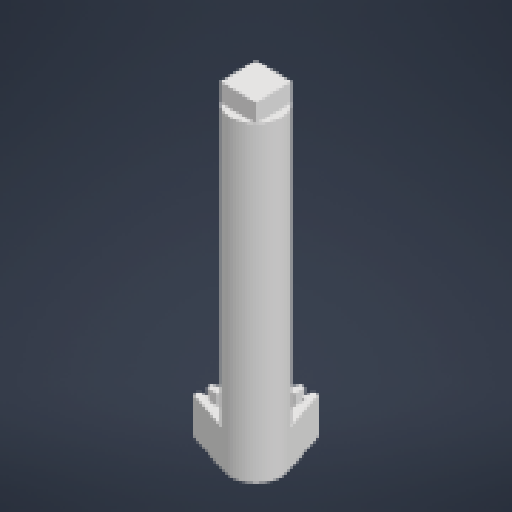
# Autodesk Inventor part: LegV2
Saved by Autodesk Inventor 2026 (Build 300175050, 175E)
## iProperties
Created: 2026-05-02
Part Number: LegV2
Material: Generic
Document SubType Name: Modeling
Designer: sniel
Density: 1 g/cm^3
Appearance: Default
Author: sniel
Autodesk Inventor part; units mm, degrees
ref_plane "YZ Plane" through (0, 0, 0) normal (1, 0, 0) x (0, 1, 0)
ref_plane "XZ Plane" through (0, 0, 0) normal (0, 1, 0) x (-1, 0, 0)
ref_plane "XY Plane" through (0, 0, 0) normal (0, 0, 1) x (1, 0, 0)
sketch "Sketch1" plane through (0, 0, 0) normal (0, 1, 0) x (-1, 0, 0)
  line L0 (0, 0) -> (10, 0)
  line L1 (0, 10) -> (0, 0)
  line L2 (10, 10) -> (0, 10)
  line L3 (10, 0) -> (10, 10)
  line L4 (0, 10) -> (0.05, 10)
  line L5 (0.05, 10) -> (0.05, 9.95)
  line L6 (0.05, 9.95) -> (0, 9.95)
  line L7 (0, 9.95) -> (0, 10)
  line L8 (10, 0) -> (9.95, 0)
  line L9 (9.95, 0) -> (9.95, 0.05)
  line L10 (9.95, 0.05) -> (10, 0.05)
  line L11 (10, 0.05) -> (10, 0)
  line L12 (0.05, 9.95) -> (9.95, 9.95)
  line L13 (9.95, 9.95) -> (9.95, 0.05)
  line L14 (9.95, 0.05) -> (0.05, 0.05)
  line L15 (0.05, 0.05) -> (0.05, 9.95)
  point P0 (0, 0)
  dimension "d0" = 0.05
  dimension "d1" = 0.05
  dimension "d2" = 0.05
  dimension "d3" = 0.05
  constraints: 32 end point, 6 parallel, 3 horizontal, 3 perpendicular
  measures "d0" distance of L5.end L6.end
  measures "d1" distance of L4.end L5.end
  measures "d2" distance of L9.end L10.end
  measures "d3" distance of L8.end L9.end
extrude "Extrusion1" add sketch "Sketch1" along normal blind 5 contours L14 L15 L12 L13
sketch "Sketch2" plane through (0, 0, 0) normal (0, -1, 0) x (1, 0, 0)
  line L0 (-0.05, 0.05) -> (-9.95, 0.05)
  line L1 (-0.05, 9.95) -> (-0.05, 0.05)
  line L2 (-9.95, 9.95) -> (-0.05, 9.95)
  line L3 (-9.95, 0.05) -> (-9.95, 9.95)
  line L4 (-0.05, 5) -> (-9.95, 5)
  circle A0 centre (-5, 5) radius 7.0004
  point P0 (0, 0)
  constraints: 10 end point, 3 midpoint, 3 other
extrude "Extrusion2" add sketch "Sketch2" along normal blind 85
sketch "Sketch4" plane through (-5, -85, 5) normal (0, -1, 0) x (1, 0, 0)
  circle A0 centre (0, 0) radius 7.0004
  circle A1 centre (0, 0) radius 7.0004 projected
  line L0 (0, -7.0004) -> (0, -12)
  line L1 (-2.5, -9.5) -> (2.5, -9.5)
  line L2 (2.5, -9.5) -> (2.5, -14.5)
  line L3 (2.5, -14.5) -> (-2.5, -14.5)
  line L4 (-2.5, -14.5) -> (-2.5, -9.5)
  line L5 (-2.5, -9.5) -> (2.5, -14.5) construction
  line L6 (2.5, -9.5) -> (-2.5, -14.5) construction
  line L7 (-7.0004, 0.0004) -> (-12.0004, 0.0004)
  line L8 (-9.5004, 2.5004) -> (-14.5004, 2.5004)
  line L9 (-14.5004, 2.5004) -> (-14.5004, -2.4996)
  line L10 (-14.5004, -2.4996) -> (-9.5004, -2.4996)
  line L11 (-9.5004, -2.4996) -> (-9.5004, 2.5004)
  line L12 (-9.5004, 2.5004) -> (-14.5004, -2.4996) construction
  line L13 (-14.5004, 2.5004) -> (-9.5004, -2.4996) construction
  line L14 (-9.5004, -2.4996) -> (-9.5004, -4.9996)
  line L15 (-14.5004, 2.5004) -> (-2.2357, 6.6338)
  line L16 (-14.5004, -2.4996) -> (-2.236, -6.6336)
  line L17 (-2.5, -14.5) -> (-6.6337, -2.2359)
  line L18 (2.5, -14.5) -> (6.6337, -2.2359)
  point P0 (5, -5)
  point P1 (-12.0004, 0.0004)
  point P2 (6.6337, -2.2359)
  point P3 (-2.2357, 6.6338)
  point P4 (-5.5251, -5.525)
  dimension "d16" = 5
  dimension "d17" = 5
  dimension "d18" = 5
  dimension "d19" = 5
  dimension "d20" = 5
  dimension "d21" = 2.5
  constraints: 38 end point, 6 point on circle, 4 midpoint, 4 parallel, 4 tangent, 3 horizontal, 2 perpendicular, 1 centre point, 1 vertical
  measures "d16" distance of L2.end L3.end
  measures "d17" distance of L1.end L2.end
  measures "d18" distance of L7.start L7.end
  measures "d19" distance of L10.end L9.end
  measures "d20" distance of L9.end L8.end
  measures "d21" distance of L10.end L14.end
extrude "Extrusion4" add sketch "Sketch4" against normal blind 10 contours A0 L7 L11 L8 L15 | L18 L2 L1 L0 A0 | A0 L17 L16 L14 L11 L7 | L8 L11 L10 L9 | L0 L1 L4 L17 L16 A0 | L3 L4 L1 L2 | A0 L16 L17 | L10 L14 L16
sketch "Sketch6" plane through (0, -85, 0) normal (0, -1, 0) x (1, 0, 0)
  arc A0 (1.6337, 2.7641) -> (-7.2357, 11.6338) centre (-5, 5) ccw
  line L0 (-7.2357, 11.6338) -> (-19.5004, 7.5004)
  line L1 (-19.5004, 7.5004) -> (-19.5004, 2.5004)
  line L2 (-19.5004, 2.5004) -> (-10.5251, -0.525)
  line L3 (-10.5251, -0.525) -> (-7.5, -9.5)
  line L4 (-7.5, -9.5) -> (-2.5, -9.5)
  line L5 (-2.5, -9.5) -> (1.6337, 2.7641)
  line L6 (-3, -6.5) -> (-7, -6.5)
  line L7 (-7, -6.5) -> (-7, -2.5)
  line L8 (-7, -2.5) -> (-3, -2.5)
  line L9 (-3, -2.5) -> (-3, -6.5)
  line L10 (-3, -6.5) -> (-7, -2.5) construction
  line L11 (-7, -6.5) -> (-3, -2.5) construction
  line L12 (-4, -9.5) -> (-6, -9.5)
  line L13 (-6, -9.5) -> (-6, -6.5)
  line L14 (-6, -6.5) -> (-4, -6.5)
  line L15 (-4, -6.5) -> (-4, -9.5)
  line L16 (-4, -9.5) -> (-6, -6.5) construction
  line L17 (-6, -9.5) -> (-4, -6.5) construction
  line L18 (-10.5251, -0.525) -> (-0.05, 9.95)
  line L19 (-10.5251, -0.525) -> (4.2889, -0.525) construction
  line L20 (-16.5004, 6.0004) -> (-19.5004, 6.0004)
  line L21 (-19.5004, 6.0004) -> (-19.5004, 4.0004)
  line L22 (-19.5004, 4.0004) -> (-16.5004, 4.0004)
  line L23 (-16.5004, 4.0004) -> (-16.5004, 6.0004)
  line L24 (-16.5004, 6.0004) -> (-19.5004, 4.0004) construction
  line L25 (-19.5004, 6.0004) -> (-16.5004, 4.0004) construction
  line L26 (-12.5004, 7.0004) -> (-16.5004, 7.0004)
  line L27 (-16.5004, 7.0004) -> (-16.5004, 3.0004)
  line L28 (-16.5004, 3.0004) -> (-12.5004, 3.0004)
  line L29 (-12.5004, 3.0004) -> (-12.5004, 7.0004)
  line L30 (-12.5004, 7.0004) -> (-16.5004, 3.0004) construction
  line L31 (-16.5004, 7.0004) -> (-12.5004, 3.0004) construction
  point P0 (0, 0)
  point P1 (-5, -8)
  dimension "d27" = 4
  dimension "d28" = 4
  dimension "d29" = 45
  dimension "d31" = 3
  dimension "d32" = 2
  dimension "d34" = 4
  dimension "d35" = 4
  constraints: 64 end point, 8 parallel, 5 horizontal, 4 perpendicular, 3 point on circle, 2 midpoint, 1 centre point, 1 equal length, 1 point on line
  measures "d27" distance of L7.end L8.end
  measures "d28" distance of L6.end L7.end
  measures "d29" angle of L19 L18
  measures "d31" distance of L22.end L21.end
  measures "d32" distance of L21.end L20.end
  measures "d34" distance of L28.end L27.end
  measures "d35" distance of L27.end L26.end
extrude "Extrusion6" cut sketch "Sketch6" against normal blind 85 contours L4 L13 L6 L15 | L6 L7 L8 L9 | L20 L23 L22 L1 | L27 L26 L29 L28 L23
body "Solid1"
